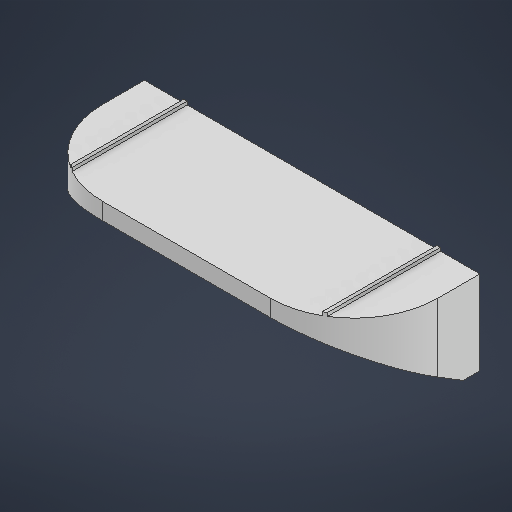
# Autodesk Inventor part: tableExtender
Saved by Autodesk Inventor 2026.3 (Build 303398000, 398)
## iProperties
Created: 2026-06-23
Part Number: tableExtender
Material: Generic
Document SubType Name: Modeling
Designer: frede
Density: 1 g/cm^3
Appearance: Default
Author: frede
Autodesk Inventor part; units mm, degrees
ref_plane "YZ Plane" through (0, 0, 0) normal (1, 0, 0) x (0, 1, 0)
ref_plane "XZ Plane" through (0, 0, 0) normal (0, 1, 0) x (-1, 0, 0)
ref_plane "XY Plane" through (0, 0, 0) normal (0, 0, 1) x (1, 0, 0)
sketch "Sketch1" plane through (0, 0, 0) normal (0, 0, 1) x (1, 0, 0)
  line L0 (0, 0) -> (200, 0)
  line L1 (200, 0) -> (200, -50)
  line L2 (200, -50) -> (0, -50)
  line L3 (0, -50) -> (0, 0)
  dimension "d0" = 200
  dimension "d1" = 50
  constraints: 8 end point, 2 parallel, 1 horizontal, 1 perpendicular
  measures "d0" distance of L1.end L2.end
  measures "d1" distance of L0.end L1.end
extrude "Extrusion1" add sketch "Sketch1" along normal blind 75
sketch "Sketch2" plane through (0, 0, 0) normal (0, 0, -1) x (-1, 0, 0)
  circle A0 centre (-175, -25) radius 7.95
  line L0 (-200, -50) -> (-200, 0) projected
  line L1 (-200, 0) -> (0, 0)
  circle A1 centre (-125, -25) radius 7.95
  circle A2 centre (-75, -25) radius 7.95
  circle A3 centre (-25, -25) radius 7.95
  dimension "d4" = 15.9
  dimension "d7" = 50
  constraints: 4 centre point, 2 end point, 2 horizontal, 6 other
  measures "d4" diameter of A0
  measures "d7" distance of A0.centre A1.centre
extrude "Extrusion2" add sketch "Sketch2" along normal blind 8
fillet "Fillet1" radius 1 4 edges at (182.95, -25, 0) (132.95, -25, 0) (82.95, -25, 0) (32.95, -25, 0)
chamfer "Chamfer1" distance 0.5 angle 45 4 edges at (182.95, -25, -8) (132.95, -25, -8) (82.95, -25, -8) (32.95, -25, -8)
sketch "Sketch3" plane through (200, -50, 0) normal (1, 0, 0) x (0, 0, -1)
  line L0 (0, 0) -> (0, 50) projected
  line L1 (0, 0) -> (-75, 0) projected
  line L2 (-75, 50) -> (-75, 40)
  line L3 (-75, 50) -> (-75, 0) projected
  line L4 (0, 0) -> (-10, 0)
  line L5 (-10, 0) -> (-75, 40)
  dimension "d18" = 10
  dimension "d19" = 10
  constraints: 6 end point, 2 point on line
  measures "d18" distance of L2.start L2.end
  measures "d19" distance of L0.start L4.end
extrude "Extrusion3" cut sketch "Sketch3" against normal up to surface (200 mm away)
sketch "Sketch4" plane through (175, -25, -8) normal (0, 0, -1) x (-1, 0, 0)
  circle A0 centre (0, 0) radius 7.95 projected
  line L0 (-25, 25) -> (175, 25) projected
  point P0 (50, 0)
  point P1 (100, 0)
  point P2 (150, 0)
  dimension "d24" = 50
  constraints: 1 coincident, 1 horizontal, 3 other
  measures "d24" distance of point (0, 0) point (50, 0)
hole "Hole1" at (175, -25, -8) at (125, -25, -8) at (75, -25, -8) at (25, -25, -8) direction (0, 0, 1) diameter 6.5 end up to surface countersink diameter 8.5 countersink angle 90
sketch "Sketch5" plane through (0, 0, 75) normal (0, 0, 1) x (1, 0, 0)
  circle A0 centre (25, -25) radius 3.25 projected
  circle A1 centre (25, -25) radius 5.25
  line L0 (200, 0) -> (0, 0) projected
  circle A2 centre (75, -25) radius 5.25
  circle A3 centre (125, -25) radius 5.25
  circle A4 centre (175, -25) radius 5.25
  dimension "d36" = 10.5
  dimension "d39" = 50
  constraints: 4 centre point, 1 coincident, 1 horizontal, 6 other
  measures "d36" diameter of A1
  measures "d39" distance of A1.centre A2.centre
extrude "Extrusion4" cut sketch "Sketch5" against normal blind 70 contours A0 | A1 | A2 | A3 | A4
fillet "Fillet4" radius 50 2 edges at (200, -5, 75) (0, -5, 75)
sketch "Sketch6" plane through (0, 0, 0) normal (0, 1, 0) x (1, 0, 0)
  line L0 (25.5, 0) -> (25.5, -68.5861)
  line L1 (174.5, 0) -> (174.5, -68.5861)
  line L2 (200, 0) -> (200, -25) projected
  line L3 (0, 0) -> (0, -25) projected
  arc A0 (23.5, -67.3999) -> (25.5, -68.5861) centre (50, -25) ccw
  arc A1 (174.5, -68.5861) -> (176.5, -67.3999) centre (150, -25) ccw
  line L4 (23.5, 0) -> (23.5, -67.3999)
  line L5 (176.5, 0) -> (176.5, -67.3999)
  line L6 (176.5, 0) -> (174.5, 0)
  line L7 (25.5, 0) -> (23.5, 0)
  dimension "d49" = 149
  dimension "d50" = 200
  dimension "d51" = 25.5
  dimension "d52" = 2
  dimension "d53" = 2
  constraints: 12 end point, 4 point on circle, 4 vertical, 2 centre point
  measures "d49" distance between parallel lines of L1 L0
  measures "d50" distance between parallel lines of L2 L3
  measures "d51" distance between parallel lines of L3 L0
  measures "d52" distance between parallel lines of L4 L0
  measures "d53" distance between parallel lines of L5 L1
extrude "Extrusion5" add sketch "Sketch6" along normal blind 2
equation "\"d51\" = -0.5 * d49 + 0.5 * d50"
body "Solid1"
